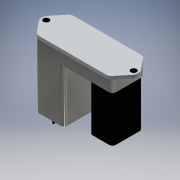
# Autodesk Inventor part: Schurter_CDG4_4101_151
Saved by Autodesk Inventor 2018 (Build 220112000, 112)
## iProperties
Created: 2013-09-03
Part Number: Schurter_CDG4_4101_151
Material: Allgemein
Document SubType Name: Modeling
Designer: strohmei
Density: 1 g/cm^3
Appearance: Schwarz
Author: strohmei
Autodesk Inventor part; units mm, degrees
ref_plane "YZ Plane" through (0, 0, 0) normal (1, 0, 0) x (0, 1, 0)
ref_plane "XZ Plane" through (0, 0, 0) normal (0, 1, 0) x (-1, 0, 0)
ref_plane "XY Plane" through (0, 0, 0) normal (0, 0, 1) x (1, 0, 0)
sketch "Skizze1" plane through (0, 0, 0) normal (0, 0, 1) x (1, 0, 0)
  line L0 (13.15, 0) -> (71.15, 0)
  line L1 (71.15, -30) -> (13.15, -30)
  arc A0 (1.7779, -11.1719) -> (1.7779, -18.8281) centre (6.398, -15) ccw
  arc A1 (82.5191, -18.827) -> (82.5191, -11.173) centre (77.898, -15) ccw
  line L2 (13.15, 0) -> (71.15, 0)
  line L3 (71.15, -30) -> (13.15, -30)
  arc A2 (13.15, 0) -> (9.6849, -1.6289) centre (13.15, -4.5) ccw
  arc A3 (9.6849, -28.3711) -> (13.15, -30) centre (13.15, -25.5) ccw
  arc A4 (71.15, -30) -> (74.6158, -28.3702) centre (71.15, -25.5) ccw
  arc A5 (74.6158, -1.6298) -> (71.15, 0) centre (71.15, -4.5) ccw
  line L4 (9.6849, -1.6289) -> (1.7779, -11.1719)
  line L5 (1.7779, -18.8281) -> (9.6849, -28.3711)
  line L6 (74.6158, -28.3702) -> (82.5191, -18.827)
  line L7 (74.6158, -1.6298) -> (82.5191, -11.173)
  line L8 (6.398, -15) -> (77.898, -15) construction
  point P0 (0, 0)
  point P1 (74.85, -30)
  dimension "d2" = 12
  dimension "d3" = 12
  dimension "d6" = 4.5
  dimension "d47" = 71.5
  dimension "d48" = 21
  dimension "d49" = 21
  dimension "d50" = 58
  dimension "d51" = 58
  dimension "d52" = 15
  dimension "d53" = 15
  dimension "d54" = 50.37
  dimension "d55" = 50.37
  dimension "d56" = 50.356
  dimension "d57" = 50.356
  constraints: 18 end point, 12 point on circle, 12 tangent, 6 centre point, 3 equal radius, 3 parallel, 3 point on line, 2 horizontal
  measures "d2" diameter of A0
  measures "d3" diameter of A1
  measures "d6" radius of A2
  measures "d47" distance of L8.end L8.start
  measures "d48" distance of A3.centre A2.centre
  measures "d49" distance of A5.centre A4.centre
  measures "d50" distance of A5.centre A2.centre
  measures "d51" distance of A3.centre A4.centre
  measures "d52" distance between parallel lines of L1 L8
  measures "d53" distance between parallel lines of L0 L8
  measures "d54" angle of L0 L7
  measures "d55" angle of L1 L6
  measures "d56" angle of L0 L4
  measures "d57" angle of L1 L5
extrude "Extrusion1" add sketch "Skizze1" against normal blind 2.8
sketch "Skizze2" plane through (0, 0, 0) normal (0, 0, 1) x (1, 0, 0)
  arc A0 (1.7779, -11.1719) -> (1.7779, -18.8281) centre (6.398, -15) ccw projected
  point P0 (0, 0)
  point P1 (4.398, -15)
  point P2 (79.898, -15)
  dimension "d9" = 75.5
  dimension "d10" = 2
  measures "d9" distance of point (79.898, -15) point (4.398, -15)
  measures "d10" distance of A0.centre point (4.398, -15)
hole "Bohrung1" at (4.398, -15, 0) at (79.898, -15, 0) direction (0, 0, -1) diameter 3.2 end through all countersink diameter 5 countersink angle 90
sketch "Skizze3" plane through (0, 0, -2.8) normal (0, 0, -1) x (-1, 0, 0)
  circle A0 centre (-79.898, -15) radius 1.6 projected
  arc A1 (-13.15, -30) -> (-9.6849, -28.3711) centre (-13.15, -25.5) ccw projected
  line L0 (-16.4119, -28.6) -> (-15.1466, -28.6)
  line L1 (-15.1466, -1.4) -> (-29.2653, -1.4)
  line L2 (-72.548, -29.1) -> (-11.748, -29.1)
  line L3 (-8.648, -26) -> (-8.648, -4)
  line L4 (-11.748, -0.9) -> (-72.548, -0.9)
  line L5 (-75.648, -4) -> (-75.648, -26)
  arc A2 (-75.648, -26) -> (-72.548, -29.1) centre (-72.548, -26) ccw
  arc A3 (-72.548, -0.9) -> (-75.648, -4) centre (-72.548, -4) ccw
  arc A4 (-8.648, -4) -> (-11.748, -0.9) centre (-11.748, -4) ccw
  arc A5 (-11.748, -29.1) -> (-8.648, -26) centre (-11.748, -26) ccw
  line L6 (-13.15, -30) -> (-71.15, -30) projected
  line L7 (-71.15, 0) -> (-13.15, 0) projected
  point P0 (0, 0)
  point P1 (-8.648, -0.9)
  point P2 (-75.648, -0.9)
  dimension "d20" = 67
  dimension "d21" = 4.25
  dimension "d22" = 3.1
  dimension "d44" = 28.2
  dimension "d45" = 0.9
  dimension "d46" = 0.9
  constraints: 12 end point, 9 point on circle, 8 tangent, 4 centre point, 4 point on line, 3 equal radius, 3 parallel, 2 horizontal, 1 perpendicular
  measures "d20" distance of point (-8.648, -0.9) point (-75.648, -0.9)
  measures "d21" distance from line of A0.centre L5
  measures "d22" radius of A2
  measures "d44" distance between parallel lines of L2 L4
  measures "d45" distance between parallel lines of L4 L7
  measures "d46" distance between parallel lines of L6 L2
extrude "Extrusion2" add sketch "Skizze3" along normal blind 10 contours A2 L5 A3 L4 A4 L3 A5 L2
sketch "Skizze4" plane through (0, 0, -12.8) normal (0, 0, -1) x (-1, 0, 0)
  line L0 (-11.748, -29.1) -> (-72.548, -29.1) projected
  line L1 (-8.648, -4) -> (-8.648, -26) projected
  line L2 (-11.748, -0.9) -> (-30.548, -0.9)
  line L3 (-33.648, -4) -> (-33.648, -26)
  line L4 (-30.548, -29.1) -> (-11.748, -29.1)
  line L5 (-8.648, -26) -> (-8.648, -4)
  arc A0 (-11.748, -29.1) -> (-8.648, -26) centre (-11.748, -26) ccw
  arc A1 (-8.648, -4) -> (-11.748, -0.9) centre (-11.748, -4) ccw
  arc A2 (-30.548, -0.9) -> (-33.648, -4) centre (-30.548, -4) ccw
  arc A3 (-33.648, -26) -> (-30.548, -29.1) centre (-30.548, -26) ccw
  point P0 (0, 0)
  point P1 (-33.648, -29.1)
  dimension "d25" = 25
  dimension "d26" = 3.1
  dimension "d27" = 0
  dimension "d28" = 3.1
  constraints: 8 end point, 8 point on circle, 8 tangent, 4 centre point, 3 point on line, 2 equal radius, 2 parallel, 1 horizontal, 1 perpendicular
  measures "d25" distance between parallel lines of L5 L3
  measures "d26" radius of A0
  measures "d27" distance between parallel lines of L5 L1
  measures "d28" radius of A1
extrude "Extrusion3" add sketch "Skizze4" along normal blind 46
sketch "Skizze5" plane through (0, 0, -58.8) normal (0, 0, -1) x (-1, 0, 0)
  line L0 (-8.648, -4) -> (-8.648, -26) projected
  line L1 (-11.748, -29.1) -> (-30.548, -29.1) projected
  line L2 (-9.848, -17.5) -> (-9.048, -17.5)
  line L3 (-9.048, -17.5) -> (-9.048, -12.7)
  line L4 (-9.048, -12.7) -> (-9.848, -12.7)
  line L5 (-9.848, -12.7) -> (-9.848, -17.5)
  line L6 (-30.548, -0.9) -> (-11.748, -0.9) projected
  line L7 (-18.448, -6.9) -> (-17.648, -6.9)
  line L8 (-17.648, -6.9) -> (-17.648, -11.7)
  line L9 (-17.648, -11.7) -> (-18.448, -11.7)
  line L10 (-18.448, -11.7) -> (-18.448, -6.9)
  line L11 (-18.448, -18.3) -> (-17.648, -18.3)
  line L12 (-17.648, -18.3) -> (-17.648, -23.1)
  line L13 (-17.648, -23.1) -> (-18.448, -23.1)
  line L14 (-18.448, -23.1) -> (-18.448, -18.3)
  point P0 (0, 0)
  dimension "d31" = 0.4
  dimension "d33" = 0.8
  dimension "d35" = 4.8
  dimension "d37" = 11.6
  dimension "d62" = 0.8
  dimension "d63" = 0.8
  dimension "d64" = 4.8
  dimension "d65" = 4.8
  dimension "d66" = 6
  dimension "d67" = 6
  dimension "d68" = 0
  dimension "d69" = 9
  constraints: 24 end point, 6 parallel, 3 horizontal, 3 perpendicular
  measures "d31" distance between parallel lines of L0 L3
  measures "d33" distance of L3.end L4.end
  measures "d35" distance of L2.end L3.end
  measures "d37" distance between parallel lines of L1 L2
  measures "d62" distance between parallel lines of L8 L10
  measures "d63" distance between parallel lines of L14 L12
  measures "d64" distance between parallel lines of L13 L11
  measures "d65" distance between parallel lines of L9 L7
  measures "d66" distance between parallel lines of L1 L13
  measures "d67" distance between parallel lines of L6 L7
  measures "d68" distance between parallel lines of L12 L8
  measures "d69" distance between parallel lines of L0 L8
extrude "Extrusion4" add sketch "Skizze5" along normal blind 8
sketch "Skizze6" plane through (0, 0, -12.8) normal (0, 0, -1) x (-1, 0, 0)
  line L0 (-30.548, -29.1) -> (-72.548, -29.1) projected
  line L1 (-71.648, -1.8) -> (-57.848, -1.8)
  line L2 (-54.748, -4.9) -> (-54.748, -25.1)
  line L3 (-74.748, -25.1) -> (-74.748, -4.9)
  arc A0 (-71.648, -1.8) -> (-74.748, -4.9) centre (-71.648, -4.9) ccw
  arc A1 (-54.748, -4.9) -> (-57.848, -1.8) centre (-57.848, -4.9) ccw
  arc A2 (-57.848, -28.2) -> (-54.748, -25.1) centre (-57.848, -25.1) ccw
  arc A3 (-74.748, -25.1) -> (-71.648, -28.2) centre (-71.648, -25.1) ccw
  line L4 (-72.548, -0.9) -> (-30.548, -0.9) projected
  line L5 (-75.648, -26) -> (-75.648, -4) projected
  line L6 (-33.648, -26) -> (-33.648, -4) projected
  line L7 (-71.648, -28.2) -> (-57.848, -28.2)
  point P0 (0, 0)
  point P1 (-54.748, -29.1)
  dimension "d40" = 20
  dimension "d41" = 3.1
  dimension "d58" = 0.9
  dimension "d59" = 0.9
  dimension "d60" = 0.9
  dimension "d61" = 26.4
  constraints: 9 point on circle, 8 end point, 8 tangent, 4 centre point, 3 equal radius, 2 perpendicular, 2 point on line, 1 horizontal, 1 parallel
  measures "d40" distance between parallel lines of L2 L3
  measures "d41" radius of A0
  measures "d58" distance between parallel lines of L5 L3
  measures "d59" distance between parallel lines of L1 L4
  measures "d60" distance between parallel lines of L0 L7
  measures "d61" distance between parallel lines of L7 L1
extrude "Extrusion5" add sketch "Skizze6" along normal blind 40.2
equation "\"d2\" = d3"
